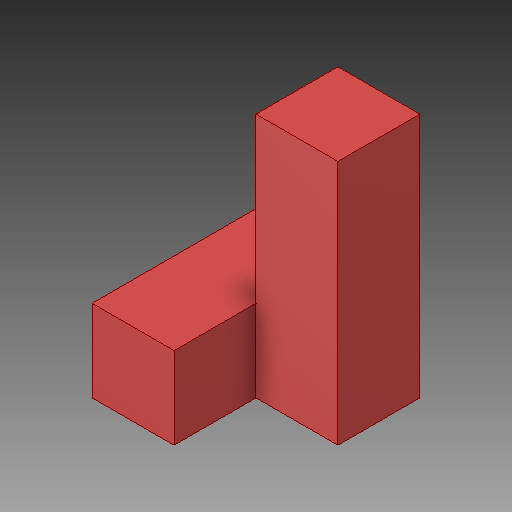
# Autodesk Inventor part: Red Part
Saved by Autodesk Inventor 2018 (Build 220112000, 112)
## iProperties
Created: 2017-11-14
Part Number: Red Part
Material: Wood (Maple)
Document SubType Name: Modeling
Designer: 232963
Density: 0.67 g/cm^3
Appearance: Smooth - Red
Mass: 23.1595 g
Surface Area: 79.8385 cm^2
Volume: 34.5665 cm^3
Author: 232963
Autodesk Inventor part; units mm, degrees
ref_plane "YZ Plane" through (0, 0, 0) normal (1, 0, 0) x (0, 1, 0)
ref_plane "XZ Plane" through (0, 0, 0) normal (0, 1, 0) x (-1, 0, 0)
ref_plane "XY Plane" through (0, 0, 0) normal (0, 0, 1) x (1, 0, 0)
sketch "Sketch1" plane through (0, 0, 0) normal (0, 0, 1) x (1, 0, 0)
  line L0 (0, 0) -> (-16.5554, 0)
  line L1 (-19.05, 19.05) -> (-19.05, 57.15)
  line L2 (-19.05, 57.15) -> (0, 57.15)
  line L3 (0, 57.15) -> (0, 0)
  line L4 (-19.05, 19.05) -> (-38.1, 19.05)
  line L5 (-38.1, 19.05) -> (-38.1, 0)
  line L6 (-38.1, 0) -> (0, 0)
  line L7 (0, 0) -> (0, 15.6896)
  dimension "d0" = 57.15
  dimension "d1" = 19.05
  dimension "d2" = 19.05
  dimension "d3" = 19.05
  constraints: 16 end point, 4 parallel, 2 horizontal, 2 perpendicular, 2 point on line
  measures "d0" distance of L2.end L0.start
  measures "d1" distance of L4.end L5.end
  measures "d2" distance of L1.start L4.end
  measures "d3" distance of L1.end L2.end
extrude "Extrusion1" add sketch "Sketch1" along normal blind 19.05
sketch "Sketch2" plane through (0, 0, 19.05) normal (0, 0, 1) x (1, 0, 0)
  line L0 (-19.05, 19.05) -> (-38.1, 19.05) projected
  line L1 (-38.1, 0) -> (0, 0) projected
  line L2 (-19.05, 19.05) -> (-38.1, 19.05)
  line L3 (-38.1, 19.05) -> (-38.1, 0)
  line L4 (-38.1, 0) -> (-19.05, 0)
  line L5 (-19.05, 0) -> (-19.05, 19.05)
  dimension "d6" = 19.05
  constraints: 8 end point, 2 parallel, 1 horizontal, 1 perpendicular
  measures "d6" distance of L4.end L0.start
extrude "Extrusion2" add sketch "Sketch2" along normal blind 19.05
body "Solid1"
